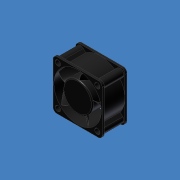
# Autodesk Inventor part: Fan-PAPST-412
Saved by Autodesk Inventor 2011 SP1 (Build 150282100, 282)
## iProperties
Shininess: 64.0
Length Units: 11272
Angle Units: 11279
Time Units: 11290
Mass Units: 11286
Length Display Precision: 3
Angle Display Precision: 2
Compacted: True
Part Number: Fan-PAPST-412
Document SubType Name: Modeling
Created: 2005-12-23
Designer: Owner
Material: ABS Plastic
Density: 1 g/cm^3
Density: 0.0
Volumn: 0.0
Area: 0.0
PropertySet Name: Model Information
Control State: 0
Master: False
Checked Out: False
Author: Owner
Autodesk Inventor part; units mm, degrees
ref_plane "YZ Plane" through (0, 0, 0) normal (1, 0, 0) x (0, 1, 0)
ref_plane "XZ Plane" through (0, 0, 0) normal (0, 1, 0) x (-1, 0, 0)
ref_plane "XY Plane" through (0, 0, 0) normal (0, 0, 1) x (1, 0, 0)
sketch "Sketch1" plane through (0, 0, 0) normal (0, 0, 1) x (1, 0, 0)
  line L0 (-19.939, 19.939) -> (19.939, 19.939)
  line L1 (19.939, 19.939) -> (19.939, -19.939)
  line L2 (19.939, -19.939) -> (-19.939, -19.939)
  line L3 (-19.939, -19.939) -> (-19.939, 19.939)
  line L4 (0, 0) -> (0, 19.939)
  line L5 (0, 0) -> (0, -19.939)
  line L6 (0, 0) -> (19.939, 0)
  line L7 (0, 0) -> (-19.939, 0)
  dimension "d0" = 39.878
  constraints: 16 end point, 4 midpoint, 3 equal length, 3 perpendicular, 2 parallel, 1 horizontal, 1 other
  measures "d0" distance of L0.start L0.end
extrude "Extrusion1" add sketch "Sketch1" along normal mid plane 20.066
sketch "Sketch2" plane through (0, 0, 0) normal (1, 0, 0) x (0, 1, 0)
  line L0 (19.939, 10.033) -> (-19.939, 10.033) projected
  line L1 (19.939, 10.033) -> (19.939, -10.033) projected
  line L2 (-19.939, -10.033) -> (19.939, -10.033) projected
  line L3 (19.939, 8.3312) -> (32.639, 8.3312)
  line L4 (32.639, 8.3312) -> (32.639, -8.3312)
  line L5 (32.639, -8.3312) -> (19.939, -8.3312)
  line L6 (0, -11.8872) -> (0, 15.8496) projected
  dimension "d3" = 1.7018
  dimension "d4" = 12.7
  dimension "d5" = 1.7018
  constraints: 6 end point, 2 perpendicular, 2 point on line, 1 parallel
  measures "d3" distance between parallel lines of L3 L0
  measures "d4" distance of L3.start L3.end
  measures "d5" distance between parallel lines of L5 L2
revolve "Revolution1" cut sketch "Sketch2" angle 360 about axis through (0, 0, -10) along (0, 0, 1) contours L3 L4 L5 L1
sketch "Sketch6" plane through (0, 0, 10.033) normal (0, 0, 1) x (1, 0, 0)
  line L0 (-19.939, 19.939) -> (19.939, 19.939) projected
  line L1 (-19.939, -19.939) -> (-19.939, 19.939) projected
  line L2 (19.939, -19.939) -> (-19.939, -19.939) projected
  line L3 (19.939, 19.939) -> (19.939, -19.939) projected
  line L4 (16.002, 16.002) -> (16.002, 19.939)
  line L5 (16.002, 16.002) -> (19.939, 16.002)
  line L6 (-16.002, -16.002) -> (-19.939, -16.002)
  line L7 (-16.002, -16.002) -> (-16.002, -19.939)
  point P0 (-16.002, 16.002)
  point P1 (16.002, -16.002)
  dimension "d28" = 32.004
  dimension "d29" = 32.004
  constraints: 8 end point, 4 point on line, 3 parallel, 3 perpendicular, 2 horizontal alignment, 2 vertical alignment
  measures "d28" distance of L6.start point (-16.002, 16.002)
  measures "d29" distance of L4.start point (-16.002, 16.002)
hole "Hole3" at (-16.002, 16.002, 10.033) at (16.002, 16.002, 10.033) at (16.002, -16.002, 10.033) at (-16.002, -16.002, 10.033) direction (0, 0, -1) diameter 4.318 end through all
sketch "Sketch7" plane through (0, 19.939, -8.3312) normal (0, 0, 1) x (1, 0, 0)
  circle A0 centre (16.002, -3.937) radius 2.159 projected
  arc A1 (19.939, -19.939) -> (0, 0) centre (0, -19.939) ccw projected
  line L0 (13.7208, -1.7286) -> (11.7128, -3.8029)
  line L1 (18.2832, -6.1454) -> (16.1928, -8.3047)
  arc A2 (18.2832, -6.1454) -> (13.7208, -1.7286) centre (16.002, -3.937) ccw
  constraints: 4 end point, 4 point on circle, 2 tangent, 1 centre point, 1 coincident, 1 parallel
extrude "Extrusion3" add sketch "Sketch7" along normal up to surface (16.6624 mm away)
pattern_circular "Circular Pattern2" count 4 over 360 about axis through (0, 0, -10) along (0, 0, 1) of "Extrusion3"
fillet "Fillet2" radius 3.175 8 edges at (19.939, 19.939, -9.1821) (19.939, 19.939, 9.1821) (-19.939, 19.939, 9.1821) (-19.939, 19.939, -9.1821) (19.939, -19.939, 9.1821) (19.939, -19.939, -9.1821) (-19.939, -19.939, 9.1821) (-19.939, -19.939, -9.1821)
sketch "Sketch8" plane through (0, 0, 10.033) normal (0, 0, 1) x (1, 0, 0)
  point P0 (0, 0)
hole "Hole4" at (0, 0, 10.033) direction (0, 0, -1) diameter 38.481 end through all
sketch "Sketch9" plane through (0, 0, 10.033) normal (0, 0, 1) x (1, 0, 0)
  circle A0 centre (0, 0) radius 19.2405 projected
  line L0 (19.939, 16.764) -> (19.939, -16.764) projected
  line L1 (-19.939, -16.764) -> (-19.939, 16.764) projected
  circle A1 centre (16.002, 16.002) radius 2.159 projected
  line L2 (10.2316, 16.2945) -> (-3.9361, 11.4049)
  line L3 (-7.5433, -9.4161) -> (-19.2404, -0.0454)
  line L4 (-11.1312, -4.6542) -> (-19.1583, 1.7764)
  line L5 (11.7284, 15.2526) -> (2.0058, 11.8971)
  arc A2 (-3.9361, 11.4049) -> (-11.1312, -4.6542) centre (0, 0) ccw
  line L6 (7.493, -9.4562) -> (7.493, -17.7215)
  line L7 (13.4874, -7.9239) -> (13.4874, -13.7218)
  line L8 (13.4874, -7.9239) -> (10.8467, -5.2833)
  arc A3 (-7.5433, -9.4161) -> (7.493, -9.4562) centre (0, 0) ccw
  arc A4 (10.8467, -5.2833) -> (2.0058, 11.8971) centre (0, 0) ccw
  dimension "d53" = 1.4732
  dimension "d54" = 12.446
  dimension "d55" = 5.9944
  dimension "d58" = 12.065
  dimension "d59" = 1.4732
  dimension "d60" = 135
  dimension "d61" = 12.065
  dimension "d62" = 12.065
  constraints: 14 end point, 12 point on circle, 3 centre point, 3 tangent, 2 parallel, 1 coincident
  measures "d53" distance between parallel lines of L4 L3
  measures "d54" distance between parallel lines of L0 L6
  measures "d55" distance between parallel lines of L7 L6
  measures "d58" radius of A2
  measures "d59" distance between parallel lines of L5 L2
  measures "d60" angle of L7 L8
  measures "d61" radius of A4
  measures "d62" radius of A3
extrude "Extrusion4" add sketch "Sketch9" against normal blind 3.81 contours L5 A4 L8 L7 A0 L6 A3 L3 L4 A2 L2
sketch "Sketch10" plane through (0, 0, 10.033) normal (0, 0, 1) x (1, 0, 0)
  line L0 (7.493, -9.4562) -> (7.493, -17.7215) projected
  line L1 (13.4874, -13.7218) -> (13.4874, -7.9239) projected
  line L2 (13.4874, -7.9239) -> (10.8467, -5.2833) projected
  arc A0 (13.4874, -13.7218) -> (11.7284, 15.2526) centre (0, 0) ccw projected
  line L3 (16.764, -19.939) -> (-16.764, -19.939) projected
  line L4 (-19.939, -16.764) -> (-19.939, 16.764) projected
  circle A1 centre (0, 0) radius 12.065
  line L5 (8.509, -8.5534) -> (8.509, -18.923)
  line L6 (8.509, -18.923) -> (12.4714, -18.923)
  line L7 (12.4714, -18.923) -> (12.4714, -8.3448)
  line L8 (12.4714, -8.3448) -> (10.3413, -6.2147)
  dimension "d65" = 1.016
  dimension "d66" = 1.016
  dimension "d67" = 1.016
  dimension "d68" = 1.016
  constraints: 8 end point, 3 parallel, 3 point on circle, 1 centre point, 1 coincident, 1 perpendicular
  measures "d65" distance between parallel lines of L5 L0
  measures "d66" distance between parallel lines of L3 L6
  measures "d67" distance between parallel lines of L7 L1
  measures "d68" distance between parallel lines of L2 L8
extrude "Extrusion5" cut sketch "Sketch10" against normal blind 2.032 contours A1 L8 L7 L6 L5
sketch "Sketch11" plane through (-16.764, -19.939, 10.033) normal (0, -1, 0) x (1, 0, 0)
  line L0 (16.764, -1.7018) -> (33.528, -1.7018) projected
  line L1 (33.528, 0) -> (0, 0) projected
  line L2 (26.7081, -1.7018) -> (27.8003, -1.7018)
  line L3 (27.8003, -1.7018) -> (27.8003, 0)
  line L4 (27.8003, 0) -> (26.7081, 0)
  line L5 (26.7081, 0) -> (26.7081, -1.7018)
  line L6 (25.273, 0) -> (25.273, -1.7018) projected
  line L7 (29.2354, 0) -> (29.2354, -1.7018) projected
  line L8 (26.7081, 0) -> (25.273, 0)
  line L9 (27.8003, 0) -> (29.2354, 0)
  dimension "d71" = 1.0922
  constraints: 12 end point, 3 collinear, 2 parallel, 2 point on line, 1 horizontal, 1 perpendicular
  measures "d71" distance between parallel lines of L3 L5
extrude "Extrusion6" cut sketch "Sketch11" against normal blind 2.54 contours L5 L1 L3 L0
sketch "Sketch12" plane through (0, 0, 6.223) normal (0, 0, -1) x (-1, 0, 0)
  arc A0 (19.2404, -0.0454) -> (19.1583, 1.7764) centre (0, 0) ccw projected
  circle A1 centre (0, 0) radius 11.938
  dimension "d74" = 23.876
  constraints: 1 centre point, 1 coincident, 1 concentric
  measures "d74" diameter of A1
extrude "Extrusion7" add sketch "Sketch12" along normal blind 16.256
fillet "Fillet3" radius 0.7874 1 edges at (11.938, 0, -10.033)
ref_plane "Work Plane1" through (0, 0, -9.271) normal (0, 0, -1) x (-1, 0, 0)
sketch "Sketch13" plane through (0, 0, -9.271) normal (0, 0, -1) x (-1, 0, 0)
  line L0 (0, 0) -> (4.0003, 18.82) construction
  line L1 (0, 0) -> (0, 19.2405) construction
  line L2 (0, 0) -> (1.3421, 19.1936) construction
  arc A0 (3.8815, 18.261) -> (3.5721, 18.3241) centre (0, 0) ccw
  arc A1 (3.8815, 18.261) -> (0.7778, 11.1234) centre (9.9705, 11.3697) ccw
  arc A2 (3.5721, 18.3241) -> (0.5234, 11.1383) centre (9.9705, 11.3697) ccw
  arc A3 (0.7778, 11.1234) -> (0.5234, 11.1383) centre (0, 0) ccw
  dimension "d83" = 4
  dimension "d84" = 12
  dimension "d85" = 37.338
  dimension "d86" = 0.254
  constraints: 8 point on circle, 6 end point, 4 centre point, 2 coincident, 2 point on line, 1 vertical
  measures "d83" angle of L2 L1
  measures "d84" angle of L0 L1
  measures "d85" diameter of A0
  measures "d86" radial gap between concentric circles of A2 A1
coil "Coil2" sketch "Sketch13" operation add axis through (0, 0, -10) along (0, 0, 1) pitch 93.1333 turns 0.15 hand right
pattern_circular "Circular Pattern4" count 5 over 360 about axis through (0, 0, -10) along (0, 0, 1) of "Coil2"
body "Solid1"
